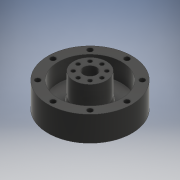
# Autodesk Inventor part: CS01
Saved by Autodesk Inventor 2017 (Build 210142000, 142)
## iProperties
Created: 2019-11-06
Part Number: CS01
Material: ABS Plastic
Document SubType Name: Modeling
Designer: Dell
Density: 1.06 g/cm^3
Appearance: Smooth - Black
Author: Dell
Autodesk Inventor part; units mm, degrees
ref_plane "YZ Plane" through (0, 0, 0) normal (1, 0, 0) x (0, 1, 0)
ref_plane "XZ Plane" through (0, 0, 0) normal (0, 1, 0) x (-1, 0, 0)
ref_plane "XY Plane" through (0, 0, 0) normal (0, 0, 1) x (1, 0, 0)
sketch "Sketch1" plane through (0, 0, 0) normal (0, 0, 1) x (1, 0, 0)
  circle A0 centre (0, 0) radius 5
  circle A1 centre (0, 0) radius 31.75
  dimension "d0" = 10
  dimension "d1" = 63.5
  constraints: 2 centre point, 2 coincident
  measures "d0" diameter of A0
  measures "d1" diameter of A1
extrude "Extrusion1" add sketch "Sketch1" along normal blind 5
sketch "Sketch2" plane through (0, 0, 5) normal (0, 0, 1) x (1, 0, 0)
  circle A0 centre (0, 0) radius 24
  circle A1 centre (0, 0) radius 31.75 projected
  dimension "d4" = 48
  constraints: 1 centre point, 1 coincident
  measures "d4" diameter of A0
extrude "Extrusion2" add sketch "Sketch2" along normal blind 14
sketch "Sketch3" plane through (0, 0, 5) normal (0, 0, 1) x (1, 0, 0)
  circle A0 centre (0, 0) radius 12.5
  circle A1 centre (0, 0) radius 5 projected
  dimension "d7" = 25
  constraints: 1 centre point, 1 coincident
  measures "d7" diameter of A0
extrude "Extrusion3" add sketch "Sketch3" along normal blind 20
chamfer "Chamfer1" distance 4 angle 15 1 edges at (-12.5, 0, 5) measured on face at (-12.5, 0, 5.5)
sketch "Sketch4" plane through (0, 0, 25) normal (0, 0, 1) x (1, 0, 0)
  circle A0 centre (9, 0) radius 1.5
  circle A1 centre (6.364, 6.364) radius 1.5
  circle A2 centre (0, 9) radius 1.5
  circle A3 centre (-6.364, 6.364) radius 1.5
  circle A4 centre (-9, 0) radius 1.5
  circle A5 centre (-6.364, -6.364) radius 1.5
  circle A6 centre (0, -9) radius 1.5
  circle A7 centre (6.364, -6.364) radius 1.5
  point P0 (0, 0)
  dimension "d13" = 3
  dimension "d14" = 9
  dimension "d17" = 360
  constraints: 8 centre point, 1 horizontal alignment, 17 other
  measures "d13" diameter of A0
  measures "d14" distance of A0.centre point (0, 0)
extrude "Extrusion4" cut sketch "Sketch4" against normal through all
sketch "Sketch5" plane through (0, 0, 19) normal (0, 0, 1) x (1, 0, 0)
  circle A0 centre (28, 0) radius 2
  circle A1 centre (19.799, 19.799) radius 2
  circle A2 centre (0, 28) radius 2
  circle A3 centre (-19.799, 19.799) radius 2
  circle A4 centre (-28, 0) radius 2
  circle A5 centre (-19.799, -19.799) radius 2
  circle A6 centre (0, -28) radius 2
  circle A7 centre (19.799, -19.799) radius 2
  point P0 (0, 0)
  dimension "d21" = 4
  dimension "d22" = 28
  dimension "d25" = 360
  constraints: 8 centre point, 1 horizontal alignment, 17 other
  measures "d21" diameter of A0
  measures "d22" distance of point (0, 0) A0.centre
extrude "Extrusion5" cut sketch "Sketch5" against normal through all
sketch "Sketch7" plane through (0, 0, 0) normal (0, 0, -1) x (-1, 0, 0)
  circle A0 centre (0, 9) radius 1.5 projected
  circle A1 centre (0, 9) radius 6.5
  circle A2 centre (0, 0) radius 15.5
  dimension "d29" = 13
  constraints: 2 centre point, 2 coincident, 1 tangent
  measures "d29" diameter of A1
extrude "Extrusion6" cut sketch "Sketch7" against normal blind 3 contours A0 | A1 | A2
body "Solid1"
